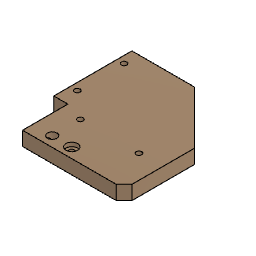
Brace BL (Autodesk Fusion 360 design; units mm, degrees)
Autodesk Fusion 360 part; units mm, degrees
sketch "Top" plane through (0, 0, 0) normal (0, 0, 1) x (1, 0, 0)
  line L0 (18, 0) -> (138.0004, 0)
  line L1 (148.0004, 10) -> (148.0004, 90)
  line L2 (80.0004, 158) -> (0, 158)
  line L3 (0, 158) -> (0, 58)
  line L4 (18, 0) -> (18, 58)
  line L5 (18, 58) -> (0, 58)
  line L6 (138.0004, 0) -> (148.0004, 10)
  line L7 (80.0004, 158) -> (148.0004, 90)
  line L8 (9, 58) -> (9, 158) construction
  line L9 (18, 49) -> (148.0004, 49) construction
  line L10 (18, 13) -> (148.0004, 13) construction
  line L11 (43, 0) -> (43, 65) construction
  circle A0 centre (9, 79) radius 3.5
  circle A1 centre (9, 139) radius 3.5
  circle A2 centre (43, 49) radius 3.5
  circle A3 centre (118, 49) radius 3.5
  circle A4 centre (43, 13) radius 6
  circle A5 centre (68, 13) radius 3.5
  circle A6 centre (68, 13) radius 7.5
  dimension "d1" = 158
  dimension "d3" = 58
  dimension "d4" = 18
  dimension "d5" = 10
  dimension "d6" = 10
  dimension "d7" = 68
  dimension "d8" = 68
  dimension "d9" = 9
  dimension "d10" = 49
  dimension "d11" = 13
  dimension "d12" = 25
  dimension "d13" = 7
  dimension "d14" = 7
  dimension "d15" = 7
  dimension "d16" = 7
  dimension "d17" = 12
  dimension "d18" = 7
  dimension "d19" = 15
  dimension "d20" = 60
  dimension "d21" = 21
  dimension "d22" = 75
  dimension "d23" = 25
  constraint horizontal L0
  constraint vertical L1
  constraint horizontal L2
  constraint vertical L3
  constraint vertical L4
  constraint horizontal L5
  constraint coincident L5 L8.start
  constraint coincident L2 L8.end
  constraint perpendicular L2 L8
  constraint coincident L4 L9.start
  constraint coincident L1 L9.end
  constraint perpendicular L1 L9
  constraint coincident L4 L10.start
  constraint coincident L1 L10.end
  constraint perpendicular L1 L10
  constraint coincident L0 L11.start
  constraint perpendicular L9 L11
  constraint coincident L8 A0.centre
  constraint coincident L8 A1.centre
  constraint coincident L11 A2.centre
  constraint coincident L9 A2.centre
  constraint coincident L9 A3.centre
  constraint coincident L10 A4.centre
  constraint coincident L11 A4.centre
  constraint coincident L10 A5.centre
  constraint concentric A5 A6
  measures "d1" distance of origin L2.end
  measures "d3" distance of origin L3.end
  measures "d4" distance of origin L0.start
  measures "d5" vertical distance of L0.end L1.start
  measures "d6" horizontal distance of L0.end L1.start
  measures "d7" vertical distance of L2.start L1.end
  measures "d8" horizontal distance of L2.start L1.end
  measures "d9" distance of L3 L8
  measures "d10" distance of L0 L9
  measures "d11" distance of L0 L10
  measures "d12" distance of L4 L11
  measures "d13" diameter of A0
  measures "d14" diameter of A1
  measures "d15" diameter of A2
  measures "d16" diameter of A3
  measures "d17" diameter of A4
  measures "d18" diameter of A5
  measures "d19" diameter of A6
  measures "d20" distance of A0.centre A1.centre
  measures "d21" distance of L5 A0.centre
  measures "d22" distance of A2.centre A3.centre
  measures "d23" distance of A4.centre A5.centre
extrude "Extrude1" add sketch "Top" along normal blind 13 contours A6
extrude "Extrude2" add sketch "Top" along normal blind 18 contours L0 L1 L2 L3 L4 L5 L6 L7
sketch "Side" plane through (18, 0, 0) normal (-1, 0, 0) x (0, -1, 0)
  line L0 (-58, 0) -> (0, 0)
  line L1 (0, 0) -> (0, 18)
  line L2 (0, 18) -> (-58, 18)
  line L3 (-58, 18) -> (-58, 0)
  line L4 (0, 0) -> (-58, 0) construction
  line L5 (-58, 0) -> (-58, 18) construction
  line L6 (-58, 18) -> (0, 18) construction
  line L7 (0, 18) -> (0, 0) construction
  line L8 (0, 9) -> (-58, 9) construction
  circle A0 centre (-13, 9) radius 3.5
  dimension "d28" = 7
  dimension "d29" = 13
  constraint horizontal L4
  constraint vertical L5
  constraint horizontal L6
  constraint vertical L7
  constraint coincident L2.end L3.start
  constraint coincident L0.end L1.start
  constraint midpoint L1 L8.start
  constraint midpoint L3 L8.end
  constraint coincident L8 A0.centre
  measures "d28" diameter of A0
  measures "d29" distance of L8.start A0.centre
extrude "Extrude3" cut sketch "Side" against normal blind 35 contours A0
named bodies: "Brace BL"
